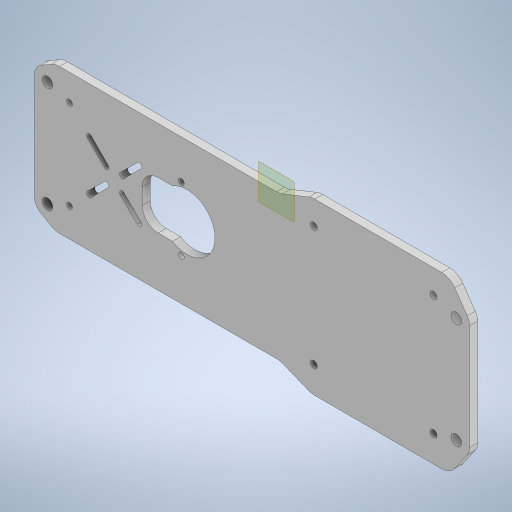
# Autodesk Inventor part: C:\Users\Kosuke\MyDrive\University\Lab\TA\3Ddata\main_frame.stp
Saved by Autodesk Inventor 2024 (Build 280153000, 153)
## iProperties
Created: 2022-08-08
Material: Generic
Document SubType Name: Modeling
Designer: OKUDA
Density: 1 g/cm^3
Appearance: Default
Sending System: Mastercam X8 ... CNC Software, Inc.
Preprocessor: STEP Write
Title: C:\Users\Kosuke\MyDrive\University\Lab\TA\3Ddata\main_frame.stp
Autodesk Inventor part; units mm, degrees
ref_plane "YZ Plane" through (0, 0, 0) normal (1, 0, 0) x (0, 1, 0)
ref_plane "XZ Plane" through (0, 0, 0) normal (0, 1, 0) x (-1, 0, 0)
ref_plane "XY Plane" through (0, 0, 0) normal (0, 0, 1) x (1, 0, 0)
ref_plane "作業平面1" through (15.3757, 45.25, -5) normal (0, 0, -1) x (-1, 0, 0)
sketch "Base_plate" plane through (15.3757, 45.25, -5) normal (0, 0, -1) x (-1, 0, 0)
  circle A0 centre (-112.6243, -12.25) radius 3.25
  circle A1 centre (-112.6243, -78.25) radius 3.25
  circle A2 centre (143.3757, -78.25) radius 3.25
  circle A3 centre (143.3757, -12.25) radius 3.25
  line L0 (151.578, -11.3644) -> (151.578, -77.3644)
  arc A4 (151.578, -11.3644) -> (147.5007, -5.1053) centre (143.3757, -12.25) ccw
  line L1 (147.5007, -5.1053) -> (140.9785, -1.3397)
  arc A5 (140.9785, -1.3397) -> (135.9785, 0) centre (135.9785, -10) ccw
  line L2 (135.9785, 0) -> (0, 0)
  line L3 (-20.2421, 7.2915) -> (-3.697, 0.7085)
  line L4 (-23.9391, 8) -> (-103.3743, 8)
  line L5 (0, 0) -> (135.9785, 0)
  arc A6 (140.9785, -1.3397) -> (135.9785, 0) centre (135.9785, -10) ccw
  line L6 (140.9785, -1.3397) -> (147.5007, -5.1053)
  arc A7 (151.578, -11.3644) -> (147.5007, -5.1053) centre (143.3757, -12.25) ccw
  line L7 (151.578, -11.3644) -> (151.578, -77.3644)
  arc A8 (147.5007, -85.3947) -> (151.578, -77.3644) centre (143.3757, -78.25) ccw
  arc A9 (-103.3743, 8) -> (-111.5876, 3.7046) centre (-103.3743, -2) ccw
  line L8 (-103.3743, 8) -> (-23.9391, 8)
  arc A10 (-20.2421, 7.2915) -> (-23.9391, 8) centre (-23.9391, -2) ccw
  line L9 (-20.2421, 7.2915) -> (-3.697, 0.7085)
  arc A11 (-3.697, 0.7085) -> (0, 0) centre (0, 10) ccw
  circle A12 centre (-112.6243, -12.25) radius 3.25
  circle A13 centre (143.3757, -12.25) radius 3.25
  circle A14 centre (143.3757, -78.25) radius 3.25
  circle A15 centre (-112.6243, -78.25) radius 3.25
  line L10 (135.9785, 0) -> (0, 0)
  arc A16 (140.9785, -1.3397) -> (135.9785, 0) centre (135.9785, -10) ccw
  line L11 (147.5007, -5.1053) -> (140.9785, -1.3397)
  arc A17 (151.578, -11.3644) -> (147.5007, -5.1053) centre (143.3757, -12.25) ccw
  line L12 (151.6257, -11.3644) -> (151.6257, -77.3644)
  arc A18 (147.5007, -85.3947) -> (151.578, -77.3644) centre (143.3757, -78.25) ccw
  line L13 (147.5007, -85.3947) -> (140.9785, -89.1603)
  arc A19 (135.9785, -90.5) -> (140.9785, -89.1603) centre (135.9785, -80.5) ccw
  line L14 (135.9785, -90.5) -> (0, -90.5)
  arc A20 (0, -90.5) -> (-3.697, -91.2085) centre (0, -100.5) ccw
  line L15 (-20.2421, -97.7915) -> (-3.697, -91.2085)
  arc A21 (-23.9391, -98.5) -> (-20.2421, -97.7915) centre (-23.9391, -88.5) ccw
  line L16 (-23.9391, -98.5) -> (-103.3743, -98.5)
  arc A22 (-111.5876, -94.2046) -> (-103.3743, -98.5) centre (-103.3743, -88.5) ccw
  line L17 (-111.5876, -94.2046) -> (-119.4003, -82.9563)
  arc A23 (-120.8743, -78.25) -> (-119.4003, -82.9563) centre (-112.6243, -78.25) ccw
  line L18 (-120.8743, -12.25) -> (-120.8743, -78.25)
  arc A24 (-119.4003, -7.5437) -> (-120.8743, -12.25) centre (-112.6243, -12.25) ccw
  line L19 (-111.5876, 3.7046) -> (-119.4003, -7.5437)
  line L20 (-23.9391, 8) -> (-103.3743, 8)
  arc A25 (-20.2421, 7.2915) -> (-23.9391, 8) centre (-23.9391, -2) ccw
  line L21 (-20.2421, 7.2915) -> (-3.697, 0.7085)
  arc A26 (-3.697, 0.7085) -> (0, 0) centre (0, 10) ccw
  line L22 (101.578, 7.8213) -> (101.578, -100.5) construction
  line L23 (151.6257, -44.3644) -> (-114.4175, -44.3644) construction
  circle A27 centre (56.078, -44.3644) radius 17.5 construction
  line L24 (129.578, -5.1053) -> (129.578, -82.9563) construction
  circle A28 centre (129.578, -16.3644) radius 1.75
  circle A29 centre (129.578, -72.3644) radius 1.75
  line L25 (59.578, -19.3302) -> (59.578, -75) construction
  circle A30 centre (59.578, -24.3644) radius 1.75
  circle A31 centre (59.578, -64.3644) radius 1.75
  circle A32 centre (101.578, -44.3644) radius 14.75 construction
  line L26 (101.578, -44.3644) -> (118.6401, -27.3023) construction
  line L27 (101.578, -44.3644) -> (125.7075, -44.3644) construction
  line L28 (106.5779, -39.3645) -> (117.1845, -28.7579) construction
  line L29 (107.7093, -40.4959) -> (118.3159, -29.8893)
  line L30 (116.0532, -27.6265) -> (105.4466, -38.2331)
  arc A33 (105.4466, -38.2331) -> (107.7093, -40.4959) centre (106.5779, -39.3645) ccw
  arc A34 (118.3159, -29.8893) -> (116.0532, -27.6265) centre (117.1845, -28.7579) ccw
  line L31 (84.8401, -29.8893) -> (95.4467, -40.4959)
  arc A35 (87.1028, -27.6265) -> (84.8401, -29.8893) centre (85.9714, -28.7579) ccw
  line L32 (97.7094, -38.2331) -> (87.1028, -27.6265)
  arc A36 (95.4467, -40.4959) -> (97.7094, -38.2331) centre (96.578, -39.3645) ccw
  line L33 (87.1028, -61.1024) -> (97.7094, -50.4958)
  arc A37 (84.8401, -58.8396) -> (87.1028, -61.1024) centre (85.9714, -59.971) ccw
  line L34 (95.4467, -48.233) -> (84.8401, -58.8396)
  arc A38 (97.7094, -50.4958) -> (95.4467, -48.233) centre (96.578, -49.3644) ccw
  line L35 (118.3159, -58.8396) -> (107.7093, -48.233)
  arc A39 (116.0532, -61.1024) -> (118.3159, -58.8396) centre (117.1845, -59.971) ccw
  line L36 (105.4466, -50.4958) -> (116.0532, -61.1024)
  arc A40 (107.7093, -48.233) -> (105.4466, -50.4958) centre (106.5779, -49.3644) ccw
  line L37 (65.0919, -29.3644) -> (74.078, -29.3644)
  line L38 (84.078, -39.3644) -> (84.078, -49.3644)
  line L39 (74.078, -59.3644) -> (65.0919, -59.3644)
  line L40 (65.0919, -59.3644) -> (65.0919, -29.3644) construction
  arc A41 (84.078, -39.3644) -> (74.078, -29.3644) centre (74.078, -39.3644) ccw
  arc A42 (74.078, -59.3644) -> (84.078, -49.3644) centre (74.078, -49.3644) ccw
  arc A43 (65.0919, -29.3644) -> (65.0919, -59.3644) centre (56.078, -44.3644) ccw
  line L41 (-60.8743, -12.5765) -> (-60.8743, -79.1684) construction
  line L42 (-98.3743, -6.8644) -> (-23.3743, -6.8644) construction
  line L43 (-23.3743, -6.8644) -> (-23.3743, -81.8644) construction
  line L44 (-23.3743, -81.8644) -> (-98.3743, -81.8644) construction
  line L45 (-98.3743, -81.8644) -> (-98.3743, -6.8644) construction
  line L46 (-98.3743, -6.8644) -> (-23.3743, -81.8644) construction
  line L47 (-23.3743, -6.8644) -> (-98.3743, -81.8644) construction
  circle A44 centre (-98.3743, -6.8644) radius 2.1
  circle A45 centre (-23.3743, -6.8644) radius 2.1
  circle A46 centre (-98.3743, -81.8644) radius 2.1
  circle A47 centre (-23.3743, -81.8644) radius 2.1
  point P0 (144.2396, -3.2225)
  point P1 (144.2396, -87.2775)
  point P2 (111.8812, -34.0612)
  point P3 (91.2747, -34.0612)
  point P4 (91.2747, -54.6677)
  point P5 (111.8812, -54.6677)
  point P6 (-60.8743, -44.3644)
  point P7 (-60.8743, -44.3644)
  dimension "d20" = 50
  dimension "d21" = 45.5
  dimension "d22" = 35
  dimension "d23" = 28
  dimension "d24" = 3.5
  dimension "d25" = 3.5
  dimension "d26" = 28
  dimension "d27" = 28
  dimension "d28" = 42
  dimension "d29" = 3.5
  dimension "d30" = 3.5
  dimension "d31" = 20
  dimension "d32" = 20
  dimension "d40" = 29.5
  dimension "d43" = 45
  dimension "d44" = 3.2
  dimension "d45" = 7.071
  dimension "d46" = 15
  dimension "d49" = 360
  dimension "d51" = 15
  dimension "d52" = 15
  dimension "d53" = 28
  dimension "d54" = 10
  dimension "d65" = 60
  dimension "d66" = 75
  dimension "d67" = 75
  dimension "d68" = 4.2
  dimension "d69" = 4.2
  dimension "d70" = 4.2
  dimension "d71" = 4.2
  constraints: 74 end point, 48 centre point, 40 point on circle, 14 point on line, 8 tangent, 7 horizontal, 6 coincident, 6 vertical, 5 midpoint, 5 parallel, 4 perpendicular, 1 equal length, 1 equal radius, 60 other
  measures "d20" distance between parallel lines of L22 L7
  measures "d21" distance from line of point (56.078, -44.364) L22
  measures "d22" diameter of A27
  measures "d23" distance between parallel lines of L22 L24
  measures "d24" diameter of A28
  measures "d25" diameter of A29
  measures "d26" distance from line of A28.centre L23
  measures "d27" distance from line of L23 A29.centre
  measures "d28" distance between parallel lines of L25 L22
  measures "d29" diameter of A30
  measures "d30" diameter of A31
  measures "d31" distance from line of A30.centre L23
  measures "d32" distance from line of L23 A31.centre
  measures "d40" diameter of A32
  measures "d43" angle of L27 L26
  measures "d44" diameter of A34
  measures "d45" distance of L26.start L28.start
  measures "d46" distance of L28.start L28.end
  measures "d51" distance between parallel lines of L23 L37
  measures "d52" distance between parallel lines of L39 L23
  measures "d53" distance from line of A27.centre L38
  measures "d54" radius of A41
  measures "d65" distance between parallel lines of L41 L18
  measures "d66" distance of L44.end L42.start
  measures "d67" distance of L42.start L42.end
  measures "d68" diameter of A44
  measures "d69" diameter of A45
  measures "d70" diameter of A46
  measures "d71" diameter of A47
sketch "RPLidarA1M8" plane through (15.3757, 45.25, -5) normal (0, 0, -1) x (-1, 0, 0)
  line L0 (59.578, -45.9195) -> (59.578, -117.33) construction
  circle A0 centre (59.578, -24.3644) radius 1.5
  circle A1 centre (59.578, -64.3644) radius 1.5
  line L1 (4.0197, -44.3644) -> (199.1363, -44.3644) construction
  circle A2 centre (129.578, -16.3644) radius 1.5
  line L2 (101.578, -2.732) -> (101.578, -85.9969) construction
  circle A3 centre (101.578, -44.3644) radius 35.14
  line L3 (59.578, -6.852) -> (59.578, -81.8768) construction
  circle A4 centre (129.578, -72.3644) radius 1.5
  line L4 (129.578, -10.2254) -> (129.578, -77.75) construction
  circle A5 centre (56.078, -44.3644) radius 10
  circle A6 centre (56.078, -44.3644) radius 16
  line L5 (151.6257, -44.3644) -> (-114.4175, -44.3644) construction
  line L6 (101.578, 7.8213) -> (101.578, -100.5) construction
  point P0 (15.3757, -88.1377)
  point P1 (59.578, -44.3644)
  point P2 (129.578, -43.9877)
  dimension "d1" = 3
  dimension "d2" = 3
  dimension "d5" = 20
  dimension "d6" = 3
  dimension "d10" = 70.28
  dimension "d11" = 42
  dimension "d12" = 40
  dimension "d13" = 3
  dimension "d14" = 28
  dimension "d15" = 28
  dimension "d16" = 28
  dimension "d17" = 20
  dimension "d18" = 45.5
  dimension "d19" = 32
  constraints: 10 end point, 9 point on line, 7 centre point, 4 midpoint, 4 vertical, 3 coincident, 1 horizontal
  measures "d1" diameter of A0
  measures "d2" diameter of A1
  measures "d5" distance from line of A0.centre L1
  measures "d6" diameter of A2
  measures "d10" diameter of A3
  measures "d11" distance between parallel lines of L3 L2
  measures "d12" distance of A1.centre A0.centre
  measures "d13" diameter of A4
  measures "d14" distance between parallel lines of L2 L4
  measures "d15" distance from line of L1 A2.centre
  measures "d16" distance from line of A4.centre L1
  measures "d17" diameter of A5
  measures "d18" distance from line of A5.centre L2
  measures "d19" diameter of A6
sketch "RPLidarA2M6" plane through (15.3757, 45.25, -5) normal (0, 0, -1) x (-1, 0, 0)
  line L0 (101.578, 7.8213) -> (101.578, -100.5) construction
  line L1 (151.6257, -44.3644) -> (-114.4175, -44.3644) construction
  circle A0 centre (101.578, -44.3644) radius 14.75 construction
  circle A1 centre (112.0078, -33.9346) radius 1.5
  line L2 (112.0078, -33.9346) -> (101.578, -44.3644) construction
  circle A2 centre (91.1482, -33.9346) radius 1.5
  circle A3 centre (91.1482, -54.7943) radius 1.5
  circle A4 centre (112.0078, -54.7943) radius 1.5
  dimension "d33" = 29.5
  dimension "d34" = 3
  dimension "d35" = 45
  dimension "d38" = 360
  constraints: 4 centre point, 2 end point, 2 point on line, 12 other
  measures "d34" diameter of A1
  measures "d35" angle of L1 L2
extrude "押し出し1" add sketch "Base_plate" along normal blind 5
